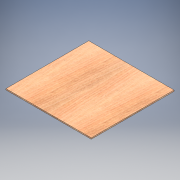
# Autodesk Inventor part: planche derrière
Saved by Autodesk Inventor 2018 (Build 220112000, 112)
## iProperties
Created: 2018-12-03
Part Number: planche derrière
Material: Wood (Birch)
Document SubType Name: Modeling
Designer: Bienvenue
Density: 0.55 g/cm^3
Appearance: Birch - Natural Polished
Author: Bienvenue
Autodesk Inventor part; units mm, degrees
ref_plane "YZ Plane" through (0, 0, 0) normal (1, 0, 0) x (0, 1, 0)
ref_plane "XZ Plane" through (0, 0, 0) normal (0, 1, 0) x (-1, 0, 0)
ref_plane "XY Plane" through (0, 0, 0) normal (0, 0, 1) x (1, 0, 0)
sketch "Sketch1" plane through (0, 0, 0) normal (0, 0, 1) x (1, 0, 0)
  line L0 (0, 0) -> (412, 0)
  line L1 (412, 0) -> (412, 412)
  line L2 (412, 412) -> (0, 412)
  line L3 (0, 412) -> (0, 0)
  dimension "d0" = 412
  dimension "d1" = 412
  constraints: 8 end point, 2 parallel, 1 horizontal, 1 perpendicular
  measures "d0" distance of L0.end L1.end
  measures "d1" distance of L1.end L2.end
extrude "Extrusion1" add sketch "Sketch1" along normal blind 6
sketch "Sketch2" plane through (0, 0, 6) normal (0, 0, 1) x (1, 0, 0)
  line L0 (412, 412) -> (0, 412) projected
  line L1 (412, 0) -> (412, 412) projected
  line L2 (0, 412) -> (412, 412)
  line L3 (412, 412) -> (412, 400)
  line L4 (412, 400) -> (0, 400)
  line L5 (0, 400) -> (0, 412)
  point P0 (0, 0)
  dimension "d4" = 12
  constraints: 8 end point, 2 parallel, 1 horizontal, 1 perpendicular, 1 point on line
  measures "d4" distance between parallel lines of L0 L4
extrude "Extrusion2" cut sketch "Sketch2" against normal blind 10
body "Solid1"
